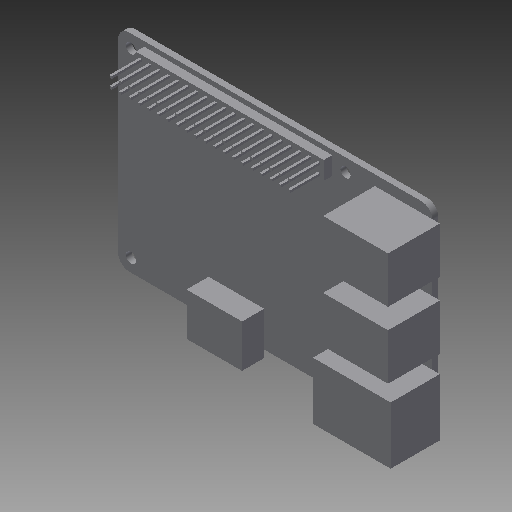
# Autodesk Inventor part: Raspberry Pi B+
Saved by Autodesk Inventor 2017 (Build 210142000, 142)
## iProperties
Created: 2014-07-27
Part Number: Raspberry Pi B+
Document SubType Name: Modeling
Designer: Nishioka
Density: 1 g/cm^3
Mass: 19.7661 g
Surface Area: 142.071 cm^2
Volume: 19.7661 cm^3
Material: 一般
Appearance: 既定
Author: Nishioka
Autodesk Inventor part; units mm, degrees
ref_plane "YZ Plane" through (0, 0, 0) normal (1, 0, 0) x (0, 1, 0)
ref_plane "XZ Plane" through (0, 0, 0) normal (0, 1, 0) x (-1, 0, 0)
ref_plane "XY Plane" through (0, 0, 0) normal (0, 0, 1) x (1, 0, 0)
sketch "スケッチ1" plane through (0, 0, 0) normal (0, 0, 1) x (1, 0, 0)
  line L0 (0, 0) -> (85, 0)
  line L1 (85, 0) -> (85, 56)
  line L2 (85, 56) -> (0, 56)
  line L3 (0, 56) -> (0, 0)
  dimension "d0" = 85
  dimension "d1" = 56
  constraints: 8 end point
  measures "d0" distance between parallel lines of L1 L3
  measures "d1" distance between parallel lines of L2 L0
extrude "押し出し1" add sketch "スケッチ1" along normal blind 1.6
sketch "スケッチ2" plane through (0, 0, 1.6) normal (0, 0, 1) x (1, 0, 0)
  line L0 (0, 0) -> (0, 56) projected
  line L1 (3.5, 52.5) -> (61.5, 52.5)
  line L2 (61.5, 52.5) -> (61.5, 3.5)
  line L3 (61.5, 3.5) -> (3.5, 3.5)
  line L4 (3.5, 3.5) -> (3.5, 52.5)
  line L5 (3.5, 28) -> (0, 28)
  dimension "d4" = 49
  dimension "d5" = 58
  dimension "d6" = 3.5
  constraints: 10 end point, 5 perpendicular, 2 midpoint
  measures "d4" distance of L3.end L1.start
  measures "d5" distance of L1.start L1.end
  measures "d6" distance between parallel lines of L0 L4
hole "穴1" at (61.5, 52.5, 1.6) at (61.5, 3.5, 1.6) at (3.5, 3.5, 1.6) at (3.5, 52.5, 1.6) direction (0, 0, -1) diameter 2.75 end through all
sketch "スケッチ3" plane through (0, 0, 1.6) normal (0, 0, 1) x (1, 0, 0)
  line L0 (85, 0) -> (0, 0) projected
  line L1 (85, 56) -> (85, 0) projected
  line L2 (69.446, 53.25) -> (87, 53.25)
  line L3 (87, 53.25) -> (87, 40.75)
  line L4 (87, 40.75) -> (69.446, 40.75)
  line L5 (69.446, 40.75) -> (69.446, 53.25)
  line L6 (87, 47) -> (81.0046, 47)
  line L7 (69.446, 35.25) -> (87, 35.25)
  line L8 (87, 35.25) -> (87, 22.75)
  line L9 (87, 22.75) -> (69.446, 22.75)
  line L10 (69.446, 22.75) -> (69.446, 35.25)
  line L11 (87, 29) -> (81.6305, 29)
  dimension "d14" = 12.5
  dimension "d15" = 2
  dimension "d16" = 17.554
  dimension "d17" = 47
  dimension "d18" = 2
  dimension "d19" = 17.554
  dimension "d20" = 12.5
  dimension "d21" = 29
  constraints: 20 end point, 6 perpendicular, 2 midpoint
  measures "d14" distance between parallel lines of L2 L4
  measures "d15" distance between parallel lines of L3 L1
  measures "d16" distance between parallel lines of L3 L5
  measures "d17" distance between parallel lines of L6 L0
  measures "d18" distance between parallel lines of L8 L1
  measures "d19" distance between parallel lines of L8 L10
  measures "d20" distance between parallel lines of L7 L9
  measures "d21" distance between parallel lines of L11 L0
extrude "押し出し2" add sketch "スケッチ3" along normal blind 14
sketch "スケッチ4" plane through (0, 0, 1.6) normal (0, 0, 1) x (1, 0, 0)
  line L0 (85, 0) -> (0, 0) projected
  line L1 (85, 22.75) -> (85, 0) projected
  line L2 (66, 18) -> (87, 18)
  line L3 (87, 18) -> (87, 2.5)
  line L4 (87, 2.5) -> (66, 2.5)
  line L5 (66, 2.5) -> (66, 18)
  line L6 (87, 10.25) -> (82.6732, 10.25)
  dimension "d24" = 2
  dimension "d26" = 21
  dimension "d27" = 10.25
  dimension "d28" = 15.5
  constraints: 10 end point, 2 perpendicular, 1 midpoint
  measures "d24" distance between parallel lines of L1 L3
  measures "d26" distance between parallel lines of L3 L5
  measures "d27" distance between parallel lines of L6 L0
  measures "d28" distance between parallel lines of L4 L2
extrude "押し出し3" add sketch "スケッチ4" along normal blind 13.3
sketch "スケッチ5" plane through (0, 0, 1.6) normal (0, 0, 1) x (1, 0, 0)
  line L0 (0, 0) -> (0, 56) projected
  line L1 (85, 0) -> (0, 0) projected
  line L2 (24.5, 9.55) -> (39.5, 9.55)
  line L3 (39.5, 9.55) -> (39.5, -2)
  line L4 (39.5, -2) -> (24.5, -2)
  line L5 (24.5, -2) -> (24.5, 9.55)
  line L6 (32, -2) -> (32, 3.163)
  dimension "d31" = 15
  dimension "d32" = 2
  dimension "d33" = 11.55
  dimension "d34" = 32
  constraints: 10 end point, 2 perpendicular, 1 midpoint
  measures "d31" distance between parallel lines of L3 L5
  measures "d32" distance between parallel lines of L1 L4
  measures "d33" distance between parallel lines of L4 L2
  measures "d34" distance between parallel lines of L6 L0
extrude "押し出し4" add sketch "スケッチ5" along normal blind 5.98
sketch "スケッチ6" plane through (0, 0, 1.6) normal (0, 0, 1) x (1, 0, 0)
  line L0 (0, 56) -> (85, 56) projected
  circle A0 centre (3.5, 52.5) radius 1.375 projected
  line L1 (7.1, 54.708) -> (57.9, 54.708)
  line L2 (57.9, 54.708) -> (57.9, 49.831)
  line L3 (57.9, 49.831) -> (7.1, 49.831)
  line L4 (7.1, 49.831) -> (7.1, 54.708)
  line L5 (32.5, 54.708) -> (32.5, 65.036)
  dimension "d37" = 29
  dimension "d38" = 4.877
  dimension "d39" = 1.292
  dimension "d40" = 50.8
  constraints: 10 end point, 4 perpendicular, 1 midpoint, 1 parallel
  measures "d37" distance from line of A0.centre L5
  measures "d38" distance between parallel lines of L1 L3
  measures "d39" distance between parallel lines of L0 L1
  measures "d40" distance between parallel lines of L2 L4
extrude "押し出し5" add sketch "スケッチ6" along normal blind 2.286 contours L1 L2 L3 L4
sketch "スケッチ7" plane through (0, 0, 3.886) normal (0, 0, 1) x (1, 0, 0)
  line L0 (7.1, 54.708) -> (57.9, 54.708) projected
  line L1 (7.1, 49.831) -> (7.1, 54.708) projected
  line L2 (8.059, 53.749) -> (8.681, 53.749)
  line L3 (8.681, 53.749) -> (8.681, 53.127)
  line L4 (8.681, 53.127) -> (8.059, 53.127)
  line L5 (8.059, 53.127) -> (8.059, 53.749)
  line L6 (8.37, 53.749) -> (8.37, 53.127)
  line L7 (8.059, 53.438) -> (8.681, 53.438)
  point P0 (0, 0)
  dimension "d43" = 0.622
  dimension "d44" = 0.622
  dimension "d45" = 1.27
  dimension "d46" = 1.27
  constraints: 12 end point, 4 midpoint, 1 perpendicular
  measures "d43" distance between parallel lines of L3 L5
  measures "d44" distance between parallel lines of L4 L2
  measures "d45" distance between parallel lines of L6 L1
  measures "d46" distance between parallel lines of L7 L0
extrude "押し出し6" add sketch "スケッチ7" along normal blind 8.077
pattern_linear "矩形状パターン1" count 2 spacing 2.54 along (0, -1, 0) count 20 spacing 2.54 along (1, 0, 0) of "押し出し6"
fillet "フィレット1" radius 3 4 edges at (85, 0, 0.8) (0, 0, 0.8) (0, 56, 0.8) (85, 56, 0.8)
